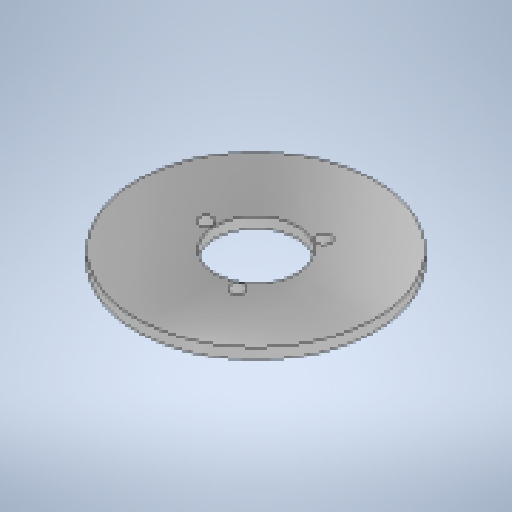
# Autodesk Inventor part: Motor Cap
Saved by Autodesk Inventor 2023.2 (Build 272271000, 271)
## iProperties
Created: 2022-12-29
Part Number: Motor Cap
Material: Aluminum 6061
Document SubType Name: Modeling
Designer: Nathan Cai
Density: 2.7 g/cm^3
Appearance: Aluminum - Flat
Author: Nathan Cai
Autodesk Inventor part; units mm, degrees
ref_plane "YZ Plane" through (0, 0, 0) normal (1, 0, 0) x (0, 1, 0)
ref_plane "XZ Plane" through (0, 0, 0) normal (0, 1, 0) x (-1, 0, 0)
ref_plane "XY Plane" through (0, 0, 0) normal (0, 0, 1) x (1, 0, 0)
sketch "Sketch1" plane through (0, 0, 0) normal (0, 1, 0) x (-1, 0, 0)
  circle A0 centre (0, 0) radius 6
  circle A1 centre (0, 0) radius 7.25 construction
  circle A2 centre (0, 0) radius 22.225 construction
  circle A3 centre (7.25, 0) radius 1
  line L0 (22.225, 0) -> (0, 0) construction
  circle A4 centre (-3.625, 6.2787) radius 1
  circle A5 centre (-3.625, -6.2787) radius 1
  circle A6 centre (0, 0) radius 17.4625
  dimension "d1" = 14.5
  dimension "d2" = 44.45
  dimension "d0" = 12
  dimension "d3" = 2
  dimension "d6" = 360
  dimension "d8" = 34.925
  constraints: 5 centre point, 4 coincident, 2 end point, 2 horizontal alignment, 1 horizontal, 1 point on line, 11 other
  measures "d0" diameter of A0
  measures "d3" diameter of A3
  measures "d8" diameter of A6
extrude "Extrusion1" add sketch "Sketch1" along normal blind 1.5875
sketch "Sketch2" plane through (0, 1.5875, 0) normal (0, 1, 0) x (1, 0, 0)
  circle A0 centre (0, 0) radius 10 construction
  line L0 (0, 0) -> (17.4625, 0) construction
  circle A1 centre (0, 0) radius 17.4625 projected
  circle A2 centre (10, 0) radius 1.7526
  circle A3 centre (-5, 8.6603) radius 1.7526
  circle A4 centre (-5, -8.6603) radius 1.7526
  dimension "d11" = 20
  dimension "d12" = 3.5052
  dimension "d15" = 360
  constraints: 3 centre point, 2 end point, 2 horizontal alignment, 1 coincident, 1 horizontal, 1 point on line, 10 other
  measures "d12" diameter of A2
extrude "Extrusion2" cut sketch "Sketch2" against normal through all contours A2 | A3 | A4
body "Solid1"
